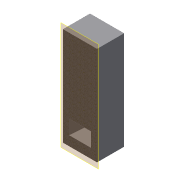
# Autodesk Inventor part: Tapered Mould
Saved by Autodesk Inventor 2015 (Build 190159000, 159)
## iProperties
Created: 2015-01-09
Part Number: Tapered Mould
Material: Generic
Document SubType Name: Modeling
Designer: jad211
Density: 1 g/cm^3
Appearance: Default
Author: jad211
Autodesk Inventor part; units mm, degrees
ref_plane "YZ Plane" through (0, 0, 0) normal (1, 0, 0) x (0, 1, 0)
ref_plane "XZ Plane" through (0, 0, 0) normal (0, 1, 0) x (-1, 0, 0)
ref_plane "XY Plane" through (0, 0, 0) normal (0, 0, 1) x (1, 0, 0)
sketch "Sketch1" plane through (0, 0, 0) normal (0, 1, 0) x (-1, 0, 0)
  line L0 (0, 0) -> (25, 0)
  line L1 (25, 0) -> (25, -72)
  line L2 (25, -72) -> (0, -72)
  line L3 (0, -72) -> (0, 0)
  dimension "d0" = 72
  dimension "d1" = 25
  constraints: 8 end point, 2 parallel, 1 horizontal, 1 perpendicular
  measures "d0" distance of L0.end L1.end
  measures "d1" distance of L1.end L2.end
extrude "Extrusion1" add sketch "Sketch1" along normal blind 25
sketch "Sketch2" plane through (0, 25, 0) normal (0, 1, 0) x (1, 0, 0)
  line L0 (-21, 5) -> (-4, 5)
  line L1 (-4, 5) -> (-4, 67)
  line L2 (-4, 67) -> (-21, 67)
  line L3 (-21, 67) -> (-21, 5)
  line L4 (-25, 72) -> (-25, 0) projected
  line L5 (0, 72) -> (-25, 72) projected
  point P0 (0, 0)
  dimension "d4" = 62
  dimension "d5" = 17
  dimension "d6" = 4
  dimension "d7" = 5
  constraints: 8 end point, 2 parallel, 1 horizontal, 1 perpendicular
  measures "d4" distance of L2.end L0.start
  measures "d5" distance of L1.end L2.end
  measures "d6" distance between parallel lines of L3 L4
  measures "d7" distance between parallel lines of L5 L2
ref_plane "Work Plane1" through (0, 5, 0) normal (0, -1, 0) x (1, 0, 0)
sketch "Sketch3" plane through (0, 5, 0) normal (0, -1, 0) x (1, 0, 0)
  line L0 (-4.5, -55) -> (-20.5, -55)
  line L1 (-20.5, -55) -> (-20.5, -65)
  line L2 (-20.5, -65) -> (-4.5, -65)
  line L3 (-4.5, -65) -> (-4.5, -55)
  line L4 (0, -72) -> (-25, -72) projected
  line L5 (0, 0) -> (0, -72) projected
  dimension "d9" = 10
  dimension "d10" = 16
  dimension "d11" = 7
  dimension "d12" = 4.5
  constraints: 8 end point, 2 parallel, 1 horizontal, 1 perpendicular
  measures "d9" distance of L2.end L0.start
  measures "d10" distance of L1.end L2.end
  measures "d11" distance between parallel lines of L4 L2
  measures "d12" distance between parallel lines of L3 L5
loft "Loft1" cut profiles "Sketch2", "Sketch3"
body "Solid1"
